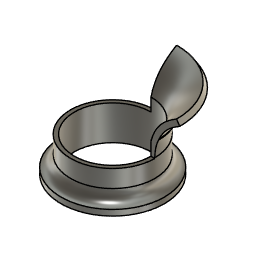
FOOD SLEEVE (Autodesk Fusion 360 design; units mm, degrees)
Autodesk Fusion 360 part; units mm, degrees
sketch "Szkic1" plane through (0, 0, 0) normal (1, 0, 0) x (0, 1, 0)
  line L0 (0, 0) -> (20, 0)
  line L1 (20, 0) -> (20, 3)
  line L2 (20, 3) -> (22, 3)
  line L3 (22, 3) -> (22, 18)
  line L4 (22, 18) -> (0, 18)
  line L5 (0, 18) -> (0, 0)
  dimension "d8" = 20
  dimension "d9" = 15
  constraint coincident L0.start L5.end
  constraint horizontal L0
  constraint perpendicular L0 L1
  constraint perpendicular L1 L2
  constraint perpendicular L2 L3
  constraint perpendicular L3 L4
  constraint perpendicular L0 L5
  measures "d8" distance of L0.start L0.end
  measures "d9" distance of L2.end L3.end
revolve "Obrót2" add sketch "Szkic1" angle 360 about axis through (0, 0, 18) along (0, 0, -1)
hole "Otwór2" at (0, 0, 0) direction (0, 0, 1) diameter 38 depth 80 tip angle 118
sketch "Szkic2" plane through (0, 0, 0) normal (1, 0, 0) x (0, 1, 0)
  line L0 (19, 18) -> (22, 18)
  line L1 (22, 18) -> (22, 28.3429)
  line L2 (23.9271, 37.2397) -> (24.3181, 38.0998)
  line L3 (32.496, 47.435) -> (35, 49)
  arc A0 (23.9271, 37.2397) -> (22, 28.3429) centre (43.5, 28.3429) ccw
  arc A1 (32.496, 47.435) -> (24.3181, 38.0998) centre (43.891, 29.203) ccw
  line L4 (19, 18) -> (19, 28.3429)
  line L5 (35, 49) -> (33.41, 51.544)
  spline S0 degree 5 poles (19, 28.3429) (19.0443, 28.9613) (19.1541, 30.1845) (19.3828, 31.979) (19.8174, 34.2895) (20.5918, 37.0314) (21.6179, 39.614) (22.9165, 42.0243) (24.4989, 44.2549) (26.3541, 46.313) (28.4616, 48.2113) (30.333, 49.6127) (31.8341, 50.602) (32.8776, 51.2345) (33.41, 51.544) knots 0 0 0 0 0 0 0.1 0.2 0.3 0.4 0.5 0.6 0.7 0.8 0.9 1 1 1 1 1 1
  point P0 (23, 42)
  dimension "d16" = 3
  constraint horizontal L0
  constraint perpendicular L0 L1
  constraint tangent L2 A0
  constraint tangent L1 A0
  constraint tangent L3 A1
  constraint tangent L2 A1
  constraint equal A0 A1
  constraint perpendicular L3 L5
  measures "d16" distance of L3.end L5.end
revolve "Obrót3" add sketch "Szkic2" angle 90 about axis through (0, 0, 1.75) along (0, 0, -1)
extrude "Wyciągnięcie proste1" add 1 faces at (7.6259, -18.4105, 18) along direction (0, 0, 1) blind 10
extrude "Wyciągnięcie proste2" cut 1 faces at (-9.2061, 17.2695, 0) along direction (0, 0, 1) blind 3
extrude "Wyciągnięcie proste3" cut 2 faces at (-2.0866, 21.177, 3) (-1.9375, 19.5215, 3) along direction (0, 0, 1) blind 10
sketch "Szkic3" plane through (0, 0, 13) normal (0, 0, -1) x (1, 0, 0)
  circle A0 centre (0, 0) radius 19
  circle A1 centre (0, 0) radius 22
  circle A2 centre (0, 0) radius 25
  circle A3 centre (0, 0) radius 20
  constraint coincident A0.centre A1.centre
extrude "Wyciągnięcie proste4" cut sketch "Szkic3" against normal blind 35 contours A3
sketch "Szkic4" plane through (0, 0, 13) normal (0, 0, -1) x (1, 0, 0)
  circle A0 centre (0, 0) radius 20
  circle A1 centre (0, 0) radius 22
  circle A2 centre (0, 0) radius 20
  circle A3 centre (0, 0) radius 27
  constraint coincident A0.centre A1.centre
  constraint concentric A2 A3
extrude "Wyciągnięcie proste5" add sketch "Szkic4" along normal blind 3 contours A1 | A3
fillet "Zaokrąglenie1" radius 6 1 edges at (7.9555, -20.5112, 13)
